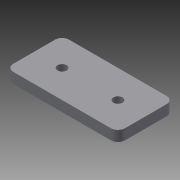
# Autodesk Inventor part: Spacer
Saved by Autodesk Inventor 2014 SP1 (Build 180222100, 222)
## iProperties
Created: 2014-01-06
Part Number: Spacer
Material: Generic
Document SubType Name: Modeling
Designer: Andrew Toennies
Density: 1 g/cm^3
Appearance: Default
Mass: 5.97413 g
Surface Area: 33.3332 cm^2
Volume: 5.97413 cm^3
Author: Andrew Toennies
Autodesk Inventor part; units mm, degrees
ref_plane "YZ Plane" through (0, 0, 0) normal (1, 0, 0) x (0, 1, 0)
ref_plane "XZ Plane" through (0, 0, 0) normal (0, 1, 0) x (-1, 0, 0)
ref_plane "XY Plane" through (0, 0, 0) normal (0, 0, 1) x (1, 0, 0)
sketch "Sketch1" plane through (0, 0, 0) normal (0, 1, 0) x (-1, 0, 0)
  line L0 (3.175, 0) -> (47.625, 0)
  line L1 (50.8, 3.175) -> (50.8, 22.225)
  line L2 (47.625, 25.4) -> (3.175, 25.4)
  line L3 (0, 22.225) -> (0, 3.175)
  arc A0 (3.175, 25.4) -> (0, 22.225) centre (3.175, 22.225) ccw
  arc A1 (0, 3.175) -> (3.175, 0) centre (3.175, 3.175) ccw
  arc A2 (47.625, 0) -> (50.8, 3.175) centre (47.625, 3.175) ccw
  arc A3 (50.8, 22.225) -> (47.625, 25.4) centre (47.625, 22.225) ccw
  point P0 (0, 0)
  point P1 (50.8, 25.4)
  point P2 (0, 25.4)
  dimension "d0" = 25.4
  dimension "d1" = 50.8
  dimension "d2" = 3.175
  constraints: 8 end point, 8 point on circle, 8 tangent, 6 point on line, 4 centre point, 3 equal radius, 2 parallel, 1 horizontal, 1 perpendicular
  measures "d0" distance of point (0, 25.4) point (0, 0)
  measures "d1" distance of point (50.8, 25.4) point (0, 25.4)
  measures "d2" radius of A0
extrude "Extrusion1" add sketch "Sketch1" along normal blind 4.7625
sketch "Sketch2" plane through (0, 4.7625, 0) normal (0, 1, 0) x (1, 0, 0)
  line L0 (-3.175, 0) -> (-47.625, 0) projected
  line L1 (-50.8, -3.175) -> (-50.8, -22.225) projected
  line L2 (-47.625, -25.4) -> (-3.175, -25.4) projected
  circle A0 centre (-38.1, -12.7) radius 2.0828
  circle A1 centre (-12.7, -12.7) radius 2.0828
  point P0 (0, 0)
  dimension "d5" = 4.1656
  dimension "d6" = 12.7
  dimension "d7" = 12.7
  dimension "d10" = 25.4
  constraints: 2 centre point, 1 horizontal, 2 other
  measures "d5" diameter of A0
  measures "d6" distance from line of L2 A0.centre
  measures "d7" distance from line of L1 A0.centre
  measures "d10" distance of A0.centre A1.centre
extrude "Extrusion2" cut sketch "Sketch2" against normal blind 4.7625
body "Solid1"
